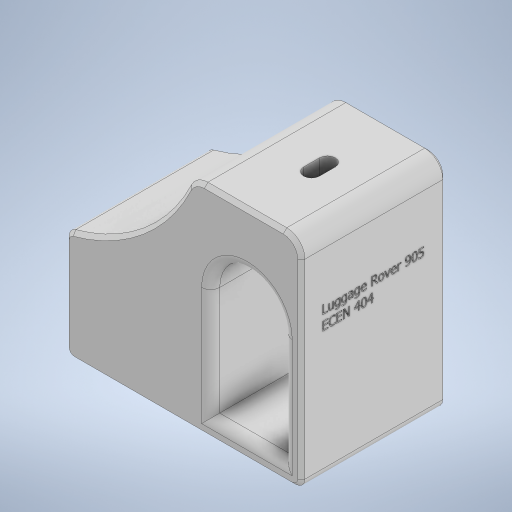
# Autodesk Inventor part: Luggage Mount
Saved by Autodesk Inventor 2023 (Build 270158000, 158)
## iProperties
Created: 2026-02-02
Part Number: Luggage Mount
Material: Generic
Document SubType Name: Modeling
Designer: Matthew
Density: 1 g/cm^3
Appearance: Default
Author: Matthew
Autodesk Inventor part; units mm, degrees
ref_plane "YZ Plane" through (0, 0, 0) normal (1, 0, 0) x (0, 1, 0)
ref_plane "XZ Plane" through (0, 0, 0) normal (0, 1, 0) x (-1, 0, 0)
ref_plane "XY Plane" through (0, 0, 0) normal (0, 0, 1) x (1, 0, 0)
sketch "Sketch1" plane through (0, 0, 0) normal (0, 0, 1) x (1, 0, 0)
  line L0 (0, 3.175) -> (0, 69.85)
  line L1 (-6.35, 76.2) -> (-19.05, 76.2)
  line L2 (-19.05, 76.2) -> (-19.05, 136.2183)
  line L3 (-19.05, 76.2) -> (-33.9583, 76.2)
  arc A0 (-80.2142, 38.6927) -> (-39.6892, 72.585) centre (-96.9975, 99.9346) ccw
  arc A1 (-33.9583, 76.2) -> (-39.6892, 72.585) centre (-33.9583, 69.85) ccw
  arc A2 (0, 69.85) -> (-6.35, 76.2) centre (-6.35, 69.85) ccw
  arc A3 (-3.175, 0) -> (0, 3.175) centre (-3.175, 3.175) ccw
  line L4 (-82.55, 35.6306) -> (-82.55, 3.175)
  line L5 (-3.175, 0) -> (-79.375, 0)
  arc A4 (-82.55, 3.175) -> (-79.375, 0) centre (-79.375, 3.175) ccw
  arc A5 (-80.2142, 38.6927) -> (-82.55, 35.6306) centre (-79.375, 35.6306) ccw
  point P0 (0, 0)
  point P1 (0, 76.2)
  point P2 (-38.1, 76.2)
  point P3 (-82.55, 38.1)
  dimension "d2" = 19.05
  dimension "d3" = 19.05
  dimension "d6" = 6.35
  dimension "d7" = 3.175
  dimension "d44" = 3.175
  constraints: 14 point on circle, 12 end point, 9 tangent, 6 centre point, 5 point on line, 3 perpendicular, 2 equal radius, 1 horizontal
  measures "d2" distance of point (0, 76.2) L1.end
  measures "d3" distance of L1.end point (-38.1, 76.2)
  measures "d6" radius of A1
  measures "d7" radius of A3
  measures "d44" radius of A4
extrude "Extrusion1" add sketch "Sketch1" along normal blind 50.8
sketch "Sketch5" plane through (0, 0, 50.8) normal (0, 0, 1) x (1, 0, 0)
  line L0 (0, 3.175) -> (0, 69.85) projected
  line L1 (0, 31.4722) -> (19.05, 31.4722) construction
  line L2 (-19.05, 0) -> (-12.7, 0) construction
  line L3 (-19.05, 6.35) -> (-6.35, 6.35)
  line L4 (-19.05, 6.35) -> (-23.1501, 6.35)
  line L5 (-19.05, 6.35) -> (-31.75, 6.35)
  line L6 (-6.35, 6.35) -> (-6.35, 44.45)
  arc A0 (-6.35, 44.45) -> (-19.05, 57.15) centre (-19.05, 44.45) ccw
  line L7 (-31.75, 44.45) -> (-31.75, 6.35)
  arc A1 (-19.05, 57.15) -> (-31.75, 44.45) centre (-19.05, 44.45) ccw
  arc A2 (-33.9583, 76.2) -> (-39.6892, 72.585) centre (-33.9583, 69.85) ccw projected
  arc A3 (-80.2142, 38.6927) -> (-39.6892, 72.585) centre (-96.9975, 99.9346) ccw projected
  arc A4 (-3.175, 0) -> (0, 3.175) centre (-3.175, 3.175) ccw projected
  line L8 (0, 3.175) -> (0, 69.85) projected
  arc A5 (0, 69.85) -> (-6.35, 76.2) centre (-6.35, 69.85) ccw projected
  line L9 (-6.35, 76.2) -> (-33.9583, 76.2) projected
  line L10 (-33.9583, 69.85) -> (-6.35, 69.85)
  line L11 (-6.35, 6.35) -> (-116.693, 6.35)
  arc A6 (-81.1052, 31.9165) -> (-116.693, 6.35) centre (-68.1025, -23.7346) ccw
  arc A7 (-80.2142, 38.6927) -> (-82.55, 35.6306) centre (-79.375, 35.6306) ccw projected
  line L12 (-82.55, 35.6306) -> (-82.55, 3.175) projected
  arc A8 (-82.55, 3.175) -> (-79.375, 0) centre (-79.375, 3.175) ccw projected
  line L13 (-79.375, 0) -> (-3.175, 0) projected
  point P0 (0, 0)
  constraints: 18 end point, 6 point on circle, 3 centre point, 3 horizontal, 1 concentric, 1 perpendicular, 1 point on line
extrude "Extrusion2" cut sketch "Sketch5" against normal blind 50.8 contours L4 L5 L7 A1 A0 L6 L3
fillet "Fillet1" radius 3.175 8 edges at (-6.35, 25.4, 50.8) (-31.75, 25.4, 50.8) (-19.05, 57.15, 50.8) (-31.75, 25.4, 0) (-6.35, 25.4, 0) (-19.05, 57.15, 0) (-19.05, 6.35, 50.8) (-19.05, 6.35, 0)
chamfer "Chamfer1" distance 1.27 angle 45 28 edges at (-20.1542, 76.2, 50.8) (-37.3462, 75.2207, 50.8) (-56.2597, 51.2244, 50.8) (-0.9299, 0.9299, 50.8) (0, 36.5125, 50.8) (-1.8599, 74.3401, 50.8) (-81.8994, 37.5563, 50.8) (-82.55, 19.4028, 50.8) (-81.6201, 0.9299, 50.8) (-41.275, 0, 50.8) (-3.175, 23.8125, 50.8) (-19.05, 3.175, 50.8) (-19.05, 60.325, 50.8) (-34.925, 23.8125, 50.8) (-20.1542, 76.2, 0) (-37.3462, 75.2207, 0) (-56.2597, 51.2244, 0) (-3.175, 23.8125, 0) (-19.05, 3.175, 0) (-19.05, 60.325, 0) (-34.925, 23.8125, 0) (-0.9299, 0.9299, 0) (0, 36.5125, 0) (-1.8599, 74.3401, 0) (-81.8994, 37.5563, 0) (-82.55, 19.4028, 0) (-81.6201, 0.9299, 0) (-41.275, 0, 0)
sketch "Sketch8" plane through (-79.375, 0, 1.27) normal (0, -1, 0) x (1, 0, 0)
  line L0 (79.375, 0) -> (79.375, 48.26) projected
  arc A0 (63.1038, 26.9088) -> (57.5462, 26.9088) centre (60.325, 26.9088) ccw
  arc A1 (57.5462, 21.3512) -> (63.1038, 21.3512) centre (60.325, 21.3512) ccw
  line L1 (57.5462, 21.3512) -> (57.5462, 26.9088)
  line L2 (63.1038, 21.3512) -> (63.1038, 26.9088)
  point P0 (79.375, -1.27)
  constraints: 4 end point, 4 point on circle, 4 tangent, 2 centre point
extrude "Extrusion4" cut sketch "Sketch8" against normal blind 25.4
sketch "Sketch9" plane through (0, 3.175, 1.27) normal (1, 0, 0) x (0, 0, -1)
  line L0 (-42.3879, 49.807) -> (-4.4919, 49.807) construction
  line L1 (-4.4919, 49.807) -> (-4.4919, 26.5095) construction
  line L2 (-4.4919, 26.5095) -> (-42.3879, 26.5095) construction
  line L3 (-42.3879, 26.5095) -> (-42.3879, 49.807) construction
  line L4 (-40.3131, 46.6973) -> (-42.0791, 46.6973)
  line L5 (-42.0791, 46.6973) -> (-42.0791, 49.7453)
  line L6 (-42.0791, 49.7453) -> (-41.6741, 49.7453)
  line L7 (-41.6741, 49.7453) -> (-41.6741, 47.0579)
  line L8 (-41.6741, 47.0579) -> (-40.3131, 47.0579)
  line L9 (-40.3131, 47.0579) -> (-40.3131, 46.6973)
  line L10 (-38.2457, 46.6973) -> (-38.631, 46.6973)
  line L11 (-38.631, 46.6973) -> (-38.631, 46.9492)
  spline S0 degree 2 poles (-38.631, 46.9492) (-38.8088, 46.7936) (-39.1275, 46.6331) (-39.3251, 46.6331) knots 0 0 0 1 2 2 2
  spline S1 degree 2 poles (-39.3251, 46.6331) (-39.4733, 46.6331) (-39.7376, 46.7319) (-39.8339, 46.8381) knots 0 0 0 1 2 2 2
  spline S2 degree 2 poles (-39.8339, 46.8381) (-39.9327, 46.9443) (-40.0414, 47.2678) (-40.0414, 47.5) knots 0 0 0 1 2 2 2
  line L12 (-40.0414, 47.5) -> (-40.0414, 48.9845)
  line L13 (-40.0414, 48.9845) -> (-39.6561, 48.9845)
  line L14 (-39.6561, 48.9845) -> (-39.6561, 47.6803)
  spline S3 degree 2 poles (-39.6561, 47.6803) (-39.6561, 47.4976) (-39.6289, 47.258) (-39.582, 47.169) knots 0 0 0 1 2 2 2
  spline S4 degree 2 poles (-39.582, 47.169) (-39.535, 47.0801) (-39.3745, 46.9986) (-39.2238, 46.9986) knots 0 0 0 1 2 2 2
  spline S5 degree 2 poles (-39.2238, 46.9986) (-39.083, 46.9986) (-38.7644, 47.1592) (-38.631, 47.2753) knots 0 0 0 1 2 2 2
  line L15 (-38.631, 47.2753) -> (-38.631, 48.9845)
  line L16 (-38.631, 48.9845) -> (-38.2457, 48.9845)
  line L17 (-38.2457, 48.9845) -> (-38.2457, 46.6973)
  spline S6 degree 2 poles (-37.6059, 46.3317) (-37.5664, 46.3144) (-37.4158, 46.2601) (-37.3194, 46.2379) knots 0 0 0 1 2 2 2
  spline S7 degree 2 poles (-37.3194, 46.2379) (-37.2132, 46.2107) (-37.0329, 46.1786) (-36.9267, 46.1786) knots 0 0 0 1 2 2 2
  spline S8 degree 2 poles (-36.9267, 46.1786) (-36.7489, 46.1786) (-36.5018, 46.2724) (-36.4327, 46.3564) knots 0 0 0 1 2 2 2
  spline S9 degree 2 poles (-36.4327, 46.3564) (-36.366, 46.4404) (-36.3141, 46.6602) (-36.3141, 46.801) knots 0 0 0 1 2 2 2
  line L18 (-36.3141, 46.801) -> (-36.3141, 47.0011)
  spline S10 degree 2 poles (-36.3141, 47.0011) (-36.4697, 46.8652) (-36.7686, 46.7368) (-36.9934, 46.7368) knots 0 0 0 1 2 2 2
  spline S11 degree 2 poles (-36.9934, 46.7368) (-37.3836, 46.7368) (-37.8455, 47.3173) (-37.8455, 47.8631) knots 0 0 0 1 2 2 2
  spline S12 degree 2 poles (-37.8455, 47.8631) (-37.8455, 48.1472) (-37.685, 48.5868) (-37.5516, 48.7424) knots 0 0 0 1 2 2 2
  spline S13 degree 2 poles (-37.5516, 48.7424) (-37.4232, 48.8882) (-37.07, 49.0487) (-36.8822, 49.0487) knots 0 0 0 1 2 2 2
  spline S14 degree 2 poles (-36.8822, 49.0487) (-36.7044, 49.0487) (-36.445, 48.9648) (-36.3141, 48.8882) knots 0 0 0 1 2 2 2
  line L19 (-36.3141, 48.8882) -> (-36.2919, 48.9845)
  line L20 (-36.2919, 48.9845) -> (-35.9288, 48.9845)
  line L21 (-35.9288, 48.9845) -> (-35.9288, 46.9591)
  spline S15 degree 2 poles (-35.9288, 46.9591) (-35.9288, 46.3762) (-36.4352, 45.8328) (-36.9563, 45.8328) knots 0 0 0 1 2 2 2
  spline S16 degree 2 poles (-36.9563, 45.8328) (-37.1243, 45.8328) (-37.475, 45.8871) (-37.6257, 45.9316) knots 0 0 0 1 2 2 2
  line L22 (-37.6257, 45.9316) -> (-37.6257, 46.3317)
  line L23 (-37.6257, 46.3317) -> (-37.6059, 46.3317)
  line L24 (-36.3141, 47.3173) -> (-36.3141, 48.5745)
  spline S17 degree 2 poles (-36.3141, 48.5745) (-36.4574, 48.6436) (-36.6995, 48.7029) (-36.8205, 48.7029) knots 0 0 0 1 2 2 2
  spline S18 degree 2 poles (-36.8205, 48.7029) (-37.1119, 48.7029) (-37.4479, 48.2731) (-37.4479, 47.8705) knots 0 0 0 1 2 2 2
  spline S19 degree 2 poles (-37.4479, 47.8705) (-37.4479, 47.4902) (-37.1935, 47.0925) (-36.9069, 47.0925) knots 0 0 0 1 2 2 2
  spline S20 degree 2 poles (-36.9069, 47.0925) (-36.7563, 47.0925) (-36.4401, 47.211) (-36.3141, 47.3173) knots 0 0 0 1 2 2 2
  spline S21 degree 2 poles (-35.2891, 46.3317) (-35.2496, 46.3144) (-35.0989, 46.2601) (-35.0025, 46.2379) knots 0 0 0 1 2 2 2
  spline S22 degree 2 poles (-35.0025, 46.2379) (-34.8963, 46.2107) (-34.716, 46.1786) (-34.6098, 46.1786) knots 0 0 0 1 2 2 2
  spline S23 degree 2 poles (-34.6098, 46.1786) (-34.432, 46.1786) (-34.185, 46.2724) (-34.1158, 46.3564) knots 0 0 0 1 2 2 2
  spline S24 degree 2 poles (-34.1158, 46.3564) (-34.0491, 46.4404) (-33.9973, 46.6602) (-33.9973, 46.801) knots 0 0 0 1 2 2 2
  line L25 (-33.9973, 46.801) -> (-33.9973, 47.0011)
  spline S25 degree 2 poles (-33.9973, 47.0011) (-34.1529, 46.8652) (-34.4517, 46.7368) (-34.6765, 46.7368) knots 0 0 0 1 2 2 2
  spline S26 degree 2 poles (-34.6765, 46.7368) (-35.0668, 46.7368) (-35.5287, 47.3173) (-35.5287, 47.8631) knots 0 0 0 1 2 2 2
  spline S27 degree 2 poles (-35.5287, 47.8631) (-35.5287, 48.1472) (-35.3681, 48.5868) (-35.2347, 48.7424) knots 0 0 0 1 2 2 2
  spline S28 degree 2 poles (-35.2347, 48.7424) (-35.1063, 48.8882) (-34.7531, 49.0487) (-34.5654, 49.0487) knots 0 0 0 1 2 2 2
  spline S29 degree 2 poles (-34.5654, 49.0487) (-34.3875, 49.0487) (-34.1282, 48.9648) (-33.9973, 48.8882) knots 0 0 0 1 2 2 2
  line L26 (-33.9973, 48.8882) -> (-33.975, 48.9845)
  line L27 (-33.975, 48.9845) -> (-33.6119, 48.9845)
  line L28 (-33.6119, 48.9845) -> (-33.6119, 46.9591)
  spline S30 degree 2 poles (-33.6119, 46.9591) (-33.6119, 46.3762) (-34.1183, 45.8328) (-34.6395, 45.8328) knots 0 0 0 1 2 2 2
  spline S31 degree 2 poles (-34.6395, 45.8328) (-34.8074, 45.8328) (-35.1582, 45.8871) (-35.3088, 45.9316) knots 0 0 0 1 2 2 2
  line L29 (-35.3088, 45.9316) -> (-35.3088, 46.3317)
  line L30 (-35.3088, 46.3317) -> (-35.2891, 46.3317)
  line L31 (-33.9973, 47.3173) -> (-33.9973, 48.5745)
  spline S32 degree 2 poles (-33.9973, 48.5745) (-34.1405, 48.6436) (-34.3826, 48.7029) (-34.5036, 48.7029) knots 0 0 0 1 2 2 2
  spline S33 degree 2 poles (-34.5036, 48.7029) (-34.7951, 48.7029) (-35.131, 48.2731) (-35.131, 47.8705) knots 0 0 0 1 2 2 2
  spline S34 degree 2 poles (-35.131, 47.8705) (-35.131, 47.4902) (-34.8766, 47.0925) (-34.5901, 47.0925) knots 0 0 0 1 2 2 2
  spline S35 degree 2 poles (-34.5901, 47.0925) (-34.4394, 47.0925) (-34.1232, 47.211) (-33.9973, 47.3173) knots 0 0 0 1 2 2 2
  spline S36 degree 2 poles (-31.7792, 46.9393) (-31.8261, 46.9048) (-31.9842, 46.7813) (-32.0583, 46.7442) knots 0 0 0 1 2 2 2
  spline S37 degree 2 poles (-32.0583, 46.7442) (-32.1596, 46.6899) (-32.3498, 46.6331) (-32.5227, 46.6331) knots 0 0 0 1 2 2 2
  spline S38 degree 2 poles (-32.5227, 46.6331) (-32.6634, 46.6331) (-32.9179, 46.7393) (-33.0142, 46.8356) knots 0 0 0 1 2 2 2
  spline S39 degree 2 poles (-33.0142, 46.8356) (-33.1056, 46.9295) (-33.2167, 47.2061) (-33.2167, 47.3592) knots 0 0 0 1 2 2 2
  spline S40 degree 2 poles (-33.2167, 47.3592) (-33.2167, 47.5964) (-33.0167, 47.9323) (-32.7993, 48.0286) knots 0 0 0 1 2 2 2
  spline S41 degree 2 poles (-32.7993, 48.0286) (-32.6066, 48.1175) (-32.083, 48.1842) (-31.7792, 48.2015) knots 0 0 0 1 2 2 2
  line L32 (-31.7792, 48.2015) -> (-31.7792, 48.2756)
  spline S42 degree 2 poles (-31.7792, 48.2756) (-31.7792, 48.409) (-31.8607, 48.5745) (-31.9348, 48.6214) knots 0 0 0 1 2 2 2
  spline S43 degree 2 poles (-31.9348, 48.6214) (-32.0089, 48.6683) (-32.2213, 48.698) (-32.3349, 48.698) knots 0 0 0 1 2 2 2
  spline S44 degree 2 poles (-32.3349, 48.698) (-32.4683, 48.698) (-32.8289, 48.6189) (-33.0092, 48.5424) knots 0 0 0 1 2 2 2
  line L33 (-33.0092, 48.5424) -> (-33.0315, 48.5424)
  line L34 (-33.0315, 48.5424) -> (-33.0315, 48.9351)
  spline S45 degree 2 poles (-33.0315, 48.9351) (-32.9253, 48.9648) (-32.5276, 49.0389) (-32.3325, 49.0389) knots 0 0 0 1 2 2 2
  spline S46 degree 2 poles (-32.3325, 49.0389) (-32.0953, 49.0389) (-31.7718, 48.9648) (-31.6433, 48.8684) knots 0 0 0 1 2 2 2
  spline S47 degree 2 poles (-31.6433, 48.8684) (-31.5174, 48.7746) (-31.3939, 48.4757) (-31.3939, 48.2608) knots 0 0 0 1 2 2 2
  line L35 (-31.3939, 48.2608) -> (-31.3939, 46.6973)
  line L36 (-31.3939, 46.6973) -> (-31.7792, 46.6973)
  line L37 (-31.7792, 46.6973) -> (-31.7792, 46.9393)
  line L38 (-31.7792, 47.2604) -> (-31.7792, 47.8952)
  spline S48 degree 2 poles (-31.7792, 47.8952) (-31.9175, 47.8829) (-32.3349, 47.8409) (-32.4658, 47.8014) knots 0 0 0 1 2 2 2
  spline S49 degree 2 poles (-32.4658, 47.8014) (-32.619, 47.7544) (-32.8191, 47.5593) (-32.8191, 47.3864) knots 0 0 0 1 2 2 2
  spline S50 degree 2 poles (-32.8191, 47.3864) (-32.8191, 47.1888) (-32.5968, 46.9887) (-32.3843, 46.9887) knots 0 0 0 1 2 2 2
  spline S51 degree 2 poles (-32.3843, 46.9887) (-32.204, 46.9887) (-31.9076, 47.1443) (-31.7792, 47.2604) knots 0 0 0 1 2 2 2
  spline S52 degree 2 poles (-30.7714, 46.3317) (-30.7319, 46.3144) (-30.5812, 46.2601) (-30.4849, 46.2379) knots 0 0 0 1 2 2 2
  spline S53 degree 2 poles (-30.4849, 46.2379) (-30.3787, 46.2107) (-30.1984, 46.1786) (-30.0922, 46.1786) knots 0 0 0 1 2 2 2
  spline S54 degree 2 poles (-30.0922, 46.1786) (-29.9143, 46.1786) (-29.6673, 46.2724) (-29.5982, 46.3564) knots 0 0 0 1 2 2 2
  spline S55 degree 2 poles (-29.5982, 46.3564) (-29.5315, 46.4404) (-29.4796, 46.6602) (-29.4796, 46.801) knots 0 0 0 1 2 2 2
  line L39 (-29.4796, 46.801) -> (-29.4796, 47.0011)
  spline S56 degree 2 poles (-29.4796, 47.0011) (-29.6352, 46.8652) (-29.9341, 46.7368) (-30.1588, 46.7368) knots 0 0 0 1 2 2 2
  spline S57 degree 2 poles (-30.1588, 46.7368) (-30.5491, 46.7368) (-31.011, 47.3173) (-31.011, 47.8631) knots 0 0 0 1 2 2 2
  spline S58 degree 2 poles (-31.011, 47.8631) (-31.011, 48.1472) (-30.8505, 48.5868) (-30.7171, 48.7424) knots 0 0 0 1 2 2 2
  spline S59 degree 2 poles (-30.7171, 48.7424) (-30.5886, 48.8882) (-30.2354, 49.0487) (-30.0477, 49.0487) knots 0 0 0 1 2 2 2
  spline S60 degree 2 poles (-30.0477, 49.0487) (-29.8699, 49.0487) (-29.6105, 48.9648) (-29.4796, 48.8882) knots 0 0 0 1 2 2 2
  line L40 (-29.4796, 48.8882) -> (-29.4574, 48.9845)
  line L41 (-29.4574, 48.9845) -> (-29.0943, 48.9845)
  line L42 (-29.0943, 48.9845) -> (-29.0943, 46.9591)
  spline S61 degree 2 poles (-29.0943, 46.9591) (-29.0943, 46.3762) (-29.6006, 45.8328) (-30.1218, 45.8328) knots 0 0 0 1 2 2 2
  spline S62 degree 2 poles (-30.1218, 45.8328) (-30.2898, 45.8328) (-30.6405, 45.8871) (-30.7912, 45.9316) knots 0 0 0 1 2 2 2
  line L43 (-30.7912, 45.9316) -> (-30.7912, 46.3317)
  line L44 (-30.7912, 46.3317) -> (-30.7714, 46.3317)
  line L45 (-29.4796, 47.3173) -> (-29.4796, 48.5745)
  spline S63 degree 2 poles (-29.4796, 48.5745) (-29.6229, 48.6436) (-29.8649, 48.7029) (-29.9859, 48.7029) knots 0 0 0 1 2 2 2
  spline S64 degree 2 poles (-29.9859, 48.7029) (-30.2774, 48.7029) (-30.6133, 48.2731) (-30.6133, 47.8705) knots 0 0 0 1 2 2 2
  spline S65 degree 2 poles (-30.6133, 47.8705) (-30.6133, 47.4902) (-30.3589, 47.0925) (-30.0724, 47.0925) knots 0 0 0 1 2 2 2
  spline S66 degree 2 poles (-30.0724, 47.0925) (-29.9217, 47.0925) (-29.6056, 47.211) (-29.4796, 47.3173) knots 0 0 0 1 2 2 2
  spline S67 degree 2 poles (-27.5431, 46.6454) (-28.0914, 46.6454) (-28.6941, 47.2604) (-28.6941, 47.8285) knots 0 0 0 1 2 2 2
  spline S68 degree 2 poles (-28.6941, 47.8285) (-28.6941, 48.3868) (-28.1087, 49.0487) (-27.637, 49.0487) knots 0 0 0 1 2 2 2
  spline S69 degree 2 poles (-27.637, 49.0487) (-27.4245, 49.0487) (-27.096, 48.9252) (-26.975, 48.7943) knots 0 0 0 1 2 2 2
  spline S70 degree 2 poles (-26.975, 48.7943) (-26.8515, 48.6634) (-26.7206, 48.2855) (-26.7206, 48.0113) knots 0 0 0 1 2 2 2
  line L46 (-26.7206, 48.0113) -> (-26.7206, 47.8014)
  line L47 (-26.7206, 47.8014) -> (-28.3039, 47.8014)
  spline S71 degree 2 poles (-28.3039, 47.8014) (-28.3039, 47.4037) (-27.9037, 46.9813) (-27.548, 46.9813) knots 0 0 0 1 2 2 2
  spline S72 degree 2 poles (-27.548, 46.9813) (-27.4221, 46.9813) (-27.1775, 47.0381) (-27.0787, 47.0826) knots 0 0 0 1 2 2 2
  spline S73 degree 2 poles (-27.0787, 47.0826) (-26.975, 47.132) (-26.8317, 47.2184) (-26.7848, 47.258) knots 0 0 0 1 2 2 2
  line L48 (-26.7848, 47.258) -> (-26.7626, 47.258)
  line L49 (-26.7626, 47.258) -> (-26.7626, 46.8381)
  spline S74 degree 2 poles (-26.7626, 46.8381) (-26.8293, 46.8109) (-27.0318, 46.7319) (-27.1108, 46.7096) knots 0 0 0 1 2 2 2
  spline S75 degree 2 poles (-27.1108, 46.7096) (-27.222, 46.6775) (-27.4048, 46.6454) (-27.5431, 46.6454) knots 0 0 0 1 2 2 2
  spline S76 degree 2 poles (-27.096, 48.0953) (-27.101, 48.2509) (-27.1652, 48.4782) (-27.2269, 48.5547) knots 0 0 0 1 2 2 2
  spline S77 degree 2 poles (-27.2269, 48.5547) (-27.2936, 48.6412) (-27.5036, 48.7326) (-27.6592, 48.7326) knots 0 0 0 1 2 2 2
  spline S78 degree 2 poles (-27.6592, 48.7326) (-27.8123, 48.7326) (-28.0272, 48.6412) (-28.1161, 48.5523) knots 0 0 0 1 2 2 2
  spline S79 degree 2 poles (-28.1161, 48.5523) (-28.2026, 48.4609) (-28.2915, 48.241) (-28.3039, 48.0953) knots 0 0 0 1 2 2 2
  line L50 (-28.3039, 48.0953) -> (-27.096, 48.0953)
  line L51 (-22.6327, 46.6973) -> (-23.1588, 46.6973)
  line L52 (-23.1588, 46.6973) -> (-24.1221, 47.9101)
  line L53 (-24.1221, 47.9101) -> (-24.5865, 47.9101)
  line L54 (-24.5865, 47.9101) -> (-24.5865, 46.6973)
  line L55 (-24.5865, 46.6973) -> (-24.9916, 46.6973)
  line L56 (-24.9916, 46.6973) -> (-24.9916, 49.7453)
  line L57 (-24.9916, 49.7453) -> (-24.2061, 49.7453)
  spline S80 degree 2 poles (-24.2061, 49.7453) (-23.9443, 49.7453) (-23.5911, 49.6885) (-23.4305, 49.5847) knots 0 0 0 1 2 2 2
  spline S81 degree 2 poles (-23.4305, 49.5847) (-23.27, 49.481) (-23.0847, 49.1574) (-23.0847, 48.9178) knots 0 0 0 1 2 2 2
  spline S82 degree 2 poles (-23.0847, 48.9178) (-23.0847, 48.5844) (-23.4256, 48.1324) (-23.717, 48.0237) knots 0 0 0 1 2 2 2
  line L58 (-23.717, 48.0237) -> (-22.6327, 46.6973)
  spline S83 degree 2 poles (-23.5071, 48.8857) (-23.5071, 49.0191) (-23.601, 49.2241) (-23.6998, 49.2908) knots 0 0 0 1 2 2 2
  spline S84 degree 2 poles (-23.6998, 49.2908) (-23.7862, 49.3476) (-24.0159, 49.3945) (-24.1839, 49.3945) knots 0 0 0 1 2 2 2
  line L59 (-24.1839, 49.3945) -> (-24.5865, 49.3945)
  line L60 (-24.5865, 49.3945) -> (-24.5865, 48.2484)
  line L61 (-24.5865, 48.2484) -> (-24.2308, 48.2484)
  spline S85 degree 2 poles (-24.2308, 48.2484) (-24.0554, 48.2484) (-23.7763, 48.3102) (-23.68, 48.4065) knots 0 0 0 1 2 2 2
  spline S86 degree 2 poles (-23.68, 48.4065) (-23.5911, 48.4905) (-23.5071, 48.7276) (-23.5071, 48.8857) knots 0 0 0 1 2 2 2
  spline S87 degree 2 poles (-20.5406, 47.8409) (-20.5406, 47.2629) (-21.0964, 46.6331) (-21.5607, 46.6331) knots 0 0 0 1 2 2 2
  spline S88 degree 2 poles (-21.5607, 46.6331) (-22.0374, 46.6331) (-22.5833, 47.2827) (-22.5833, 47.8409) knots 0 0 0 1 2 2 2
  spline S89 degree 2 poles (-22.5833, 47.8409) (-22.5833, 48.4139) (-22.0201, 49.0487) (-21.5607, 49.0487) knots 0 0 0 1 2 2 2
  spline S90 degree 2 poles (-21.5607, 49.0487) (-21.0964, 49.0487) (-20.5406, 48.4164) (-20.5406, 47.8409) knots 0 0 0 1 2 2 2
  spline S91 degree 2 poles (-20.9383, 47.8409) (-20.9383, 48.2855) (-21.2618, 48.7177) (-21.5607, 48.7177) knots 0 0 0 1 2 2 2
  spline S92 degree 2 poles (-21.5607, 48.7177) (-21.8596, 48.7177) (-22.1856, 48.2855) (-22.1856, 47.8409) knots 0 0 0 1 2 2 2
  spline S93 degree 2 poles (-22.1856, 47.8409) (-22.1856, 47.4086) (-21.8596, 46.964) (-21.5607, 46.964) knots 0 0 0 1 2 2 2
  spline S94 degree 2 poles (-21.5607, 46.964) (-21.2643, 46.964) (-20.9383, 47.4012) (-20.9383, 47.8409) knots 0 0 0 1 2 2 2
  line L62 (-18.3497, 48.9845) -> (-19.2117, 46.6973)
  line L63 (-19.2117, 46.6973) -> (-19.5575, 46.6973)
  line L64 (-19.5575, 46.6973) -> (-20.4122, 48.9845)
  line L65 (-20.4122, 48.9845) -> (-19.9947, 48.9845)
  line L66 (-19.9947, 48.9845) -> (-19.3698, 47.2234)
  line L67 (-19.3698, 47.2234) -> (-18.7498, 48.9845)
  line L68 (-18.7498, 48.9845) -> (-18.3497, 48.9845)
  spline S95 degree 2 poles (-17.0653, 46.6454) (-17.6136, 46.6454) (-18.2163, 47.2604) (-18.2163, 47.8285) knots 0 0 0 1 2 2 2
  spline S96 degree 2 poles (-18.2163, 47.8285) (-18.2163, 48.3868) (-17.6309, 49.0487) (-17.1592, 49.0487) knots 0 0 0 1 2 2 2
  spline S97 degree 2 poles (-17.1592, 49.0487) (-16.9467, 49.0487) (-16.6182, 48.9252) (-16.4972, 48.7943) knots 0 0 0 1 2 2 2
  spline S98 degree 2 poles (-16.4972, 48.7943) (-16.3737, 48.6634) (-16.2428, 48.2855) (-16.2428, 48.0113) knots 0 0 0 1 2 2 2
  line L69 (-16.2428, 48.0113) -> (-16.2428, 47.8014)
  line L70 (-16.2428, 47.8014) -> (-17.8261, 47.8014)
  spline S99 degree 2 poles (-17.8261, 47.8014) (-17.8261, 47.4037) (-17.4259, 46.9813) (-17.0702, 46.9813) knots 0 0 0 1 2 2 2
  spline S100 degree 2 poles (-17.0702, 46.9813) (-16.9443, 46.9813) (-16.6997, 47.0381) (-16.6009, 47.0826) knots 0 0 0 1 2 2 2
  spline S101 degree 2 poles (-16.6009, 47.0826) (-16.4972, 47.132) (-16.3539, 47.2184) (-16.307, 47.258) knots 0 0 0 1 2 2 2
  line L71 (-16.307, 47.258) -> (-16.2848, 47.258)
  line L72 (-16.2848, 47.258) -> (-16.2848, 46.8381)
  spline S102 degree 2 poles (-16.2848, 46.8381) (-16.3515, 46.8109) (-16.554, 46.7319) (-16.633, 46.7096) knots 0 0 0 1 2 2 2
  spline S103 degree 2 poles (-16.633, 46.7096) (-16.7442, 46.6775) (-16.927, 46.6454) (-17.0653, 46.6454) knots 0 0 0 1 2 2 2
  spline S104 degree 2 poles (-16.6182, 48.0953) (-16.6232, 48.2509) (-16.6874, 48.4782) (-16.7491, 48.5547) knots 0 0 0 1 2 2 2
  spline S105 degree 2 poles (-16.7491, 48.5547) (-16.8158, 48.6412) (-17.0258, 48.7326) (-17.1814, 48.7326) knots 0 0 0 1 2 2 2
  spline S106 degree 2 poles (-17.1814, 48.7326) (-17.3345, 48.7326) (-17.5494, 48.6412) (-17.6383, 48.5523) knots 0 0 0 1 2 2 2
  spline S107 degree 2 poles (-17.6383, 48.5523) (-17.7248, 48.4609) (-17.8137, 48.241) (-17.8261, 48.0953) knots 0 0 0 1 2 2 2
  line L73 (-17.8261, 48.0953) -> (-16.6182, 48.0953)
  line L74 (-14.6397, 48.572) -> (-14.6595, 48.572)
  spline S108 degree 2 poles (-14.6595, 48.572) (-14.704, 48.5844) (-14.8003, 48.5893) (-14.867, 48.5893) knots 0 0 0 1 2 2 2
  spline S109 degree 2 poles (-14.867, 48.5893) (-15.0226, 48.5893) (-15.3289, 48.4535) (-15.4672, 48.3201) knots 0 0 0 1 2 2 2
  line L75 (-15.4672, 48.3201) -> (-15.4672, 46.6973)
  line L76 (-15.4672, 46.6973) -> (-15.8525, 46.6973)
  line L77 (-15.8525, 46.6973) -> (-15.8525, 48.9845)
  line L78 (-15.8525, 48.9845) -> (-15.4672, 48.9845)
  line L79 (-15.4672, 48.9845) -> (-15.4672, 48.6436)
  spline S110 degree 2 poles (-15.4672, 48.6436) (-15.2572, 48.8314) (-14.9435, 48.9845) (-14.7953, 48.9845) knots 0 0 0 1 2 2 2
  spline S111 degree 2 poles (-14.7953, 48.9845) (-14.7361, 48.9845) (-14.6768, 48.9796) (-14.6397, 48.9722) knots 0 0 0 1 2 2 2
  line L80 (-14.6397, 48.9722) -> (-14.6397, 48.572)
  spline S112 degree 2 poles (-13.1725, 48.7548) (-13.1725, 48.9895) (-13.0194, 49.3797) (-12.886, 49.5205) knots 0 0 0 1 2 2 2
  spline S113 degree 2 poles (-12.886, 49.5205) (-12.7601, 49.6564) (-12.392, 49.807) (-12.2043, 49.807) knots 0 0 0 1 2 2 2
  spline S114 degree 2 poles (-12.2043, 49.807) (-11.9943, 49.807) (-11.6535, 49.6662) (-11.5275, 49.5329) knots 0 0 0 1 2 2 2
  spline S115 degree 2 poles (-11.5275, 49.5329) (-11.3694, 49.3649) (-11.1965, 48.8215) (-11.1965, 48.4041) knots 0 0 0 1 2 2 2
  spline S116 degree 2 poles (-11.1965, 48.4041) (-11.1965, 48.0261) (-11.367, 47.3494) (-11.5325, 47.1246) knots 0 0 0 1 2 2 2
  spline S117 degree 2 poles (-11.5325, 47.1246) (-11.7078, 46.8875) (-12.2018, 46.638) (-12.5625, 46.638) knots 0 0 0 1 2 2 2
  spline S118 degree 2 poles (-12.5625, 46.638) (-12.644, 46.638) (-12.8292, 46.6553) (-12.9083, 46.68) knots 0 0 0 1 2 2 2
  line L81 (-12.9083, 46.68) -> (-12.9083, 47.0727)
  line L82 (-12.9083, 47.0727) -> (-12.8885, 47.0727)
  spline S119 degree 2 poles (-12.8885, 47.0727) (-12.8366, 47.0431) (-12.6193, 46.9912) (-12.5081, 46.9912) knots 0 0 0 1 2 2 2
  spline S120 degree 2 poles (-12.5081, 46.9912) (-12.108, 46.9912) (-11.651, 47.5198) (-11.6189, 48.0089) knots 0 0 0 1 2 2 2
  spline S121 degree 2 poles (-11.6189, 48.0089) (-11.7819, 47.8977) (-12.0783, 47.7964) (-12.2537, 47.7964) knots 0 0 0 1 2 2 2
  spline S122 degree 2 poles (-12.2537, 47.7964) (-12.4217, 47.7964) (-12.7008, 47.8705) (-12.8416, 47.9767) knots 0 0 0 1 2 2 2
  spline S123 degree 2 poles (-12.8416, 47.9767) (-13.0046, 48.1027) (-13.1725, 48.4856) (-13.1725, 48.7548) knots 0 0 0 1 2 2 2
  spline S124 degree 2 poles (-11.609, 48.4954) (-11.609, 48.8042) (-11.7226, 49.1945) (-11.8239, 49.3007) knots 0 0 0 1 2 2 2
  spline S125 degree 2 poles (-11.8239, 49.3007) (-11.9128, 49.3995) (-12.0981, 49.4736) (-12.2068, 49.4736) knots 0 0 0 1 2 2 2
  spline S126 degree 2 poles (-12.2068, 49.4736) (-12.4587, 49.4736) (-12.7576, 49.113) (-12.7576, 48.7721) knots 0 0 0 1 2 2 2
  spline S127 degree 2 poles (-12.7576, 48.7721) (-12.7576, 48.5794) (-12.6588, 48.33) (-12.5501, 48.241) knots 0 0 0 1 2 2 2
  spline S128 degree 2 poles (-12.5501, 48.241) (-12.4711, 48.1768) (-12.2759, 48.1348) (-12.1623, 48.1348) knots 0 0 0 1 2 2 2
  spline S129 degree 2 poles (-12.1623, 48.1348) (-12.0314, 48.1348) (-11.7301, 48.2262) (-11.6164, 48.3028) knots 0 0 0 1 2 2 2
  spline S130 degree 2 poles (-11.6164, 48.3028) (-11.614, 48.3324) (-11.609, 48.4337) (-11.609, 48.4954) knots 0 0 0 1 2 2 2
  spline S131 degree 2 poles (-8.9044, 48.2213) (-8.9044, 47.4012) (-9.3811, 46.6331) (-9.8775, 46.6331) knots 0 0 0 1 2 2 2
  spline S132 degree 2 poles (-9.8775, 46.6331) (-10.3814, 46.6331) (-10.8532, 47.4161) (-10.8532, 48.2188) knots 0 0 0 1 2 2 2
  spline S133 degree 2 poles (-10.8532, 48.2188) (-10.8532, 49.0438) (-10.3765, 49.807) (-9.8775, 49.807) knots 0 0 0 1 2 2 2
  spline S134 degree 2 poles (-9.8775, 49.807) (-9.3761, 49.807) (-8.9044, 49.0166) (-8.9044, 48.2213) knots 0 0 0 1 2 2 2
  spline S135 degree 2 poles (-9.428, 47.2925) (-9.3687, 47.4432) (-9.3193, 47.9076) (-9.3193, 48.2213) knots 0 0 0 1 2 2 2
  spline S136 degree 2 poles (-9.3193, 48.2213) (-9.3193, 48.535) (-9.3687, 48.9969) (-9.4305, 49.1525) knots 0 0 0 1 2 2 2
  spline S137 degree 2 poles (-9.4305, 49.1525) (-9.4922, 49.3081) (-9.7071, 49.4686) (-9.8775, 49.4686) knots 0 0 0 1 2 2 2
  spline S138 degree 2 poles (-9.8775, 49.4686) (-10.048, 49.4686) (-10.2678, 49.3081) (-10.332, 49.1475) knots 0 0 0 1 2 2 2
  spline S139 degree 2 poles (-10.332, 49.1475) (-10.3938, 48.9919) (-10.4382, 48.5177) (-10.4382, 48.2188) knots 0 0 0 1 2 2 2
  spline S140 degree 2 poles (-10.4382, 48.2188) (-10.4382, 47.8977) (-10.3987, 47.4679) (-10.3345, 47.3) knots 0 0 0 1 2 2 2
  spline S141 degree 2 poles (-10.3345, 47.3) (-10.2752, 47.1419) (-10.0554, 46.9714) (-9.8775, 46.9714) knots 0 0 0 1 2 2 2
  spline S142 degree 2 poles (-9.8775, 46.9714) (-9.7096, 46.9714) (-9.4898, 47.132) (-9.428, 47.2925) knots 0 0 0 1 2 2 2
  spline S143 degree 2 poles (-6.6665, 47.6655) (-6.6665, 47.4457) (-6.8073, 47.0702) (-6.9358, 46.9319) knots 0 0 0 1 2 2 2
  spline S144 degree 2 poles (-6.9358, 46.9319) (-7.0642, 46.7936) (-7.447, 46.6331) (-7.6842, 46.6331) knots 0 0 0 1 2 2 2
  spline S145 degree 2 poles (-7.6842, 46.6331) (-7.9015, 46.6331) (-8.3264, 46.7294) (-8.482, 46.806) knots 0 0 0 1 2 2 2
  line L83 (-8.482, 46.806) -> (-8.482, 47.2382)
  line L84 (-8.482, 47.2382) -> (-8.4523, 47.2382)
  spline S146 degree 2 poles (-8.4523, 47.2382) (-8.4054, 47.2036) (-8.23, 47.1147) (-8.1238, 47.0752) knots 0 0 0 1 2 2 2
  spline S147 degree 2 poles (-8.1238, 47.0752) (-8.0028, 47.0332) (-7.8027, 46.9863) (-7.6768, 46.9863) knots 0 0 0 1 2 2 2
  spline S148 degree 2 poles (-7.6768, 46.9863) (-7.5533, 46.9863) (-7.3211, 47.0752) (-7.2371, 47.1715) knots 0 0 0 1 2 2 2
  spline S149 degree 2 poles (-7.2371, 47.1715) (-7.1605, 47.2629) (-7.0815, 47.505) (-7.0815, 47.668) knots 0 0 0 1 2 2 2
  spline S150 degree 2 poles (-7.0815, 47.668) (-7.0815, 47.831) (-7.1704, 48.0385) (-7.2544, 48.1077) knots 0 0 0 1 2 2 2
  spline S151 degree 2 poles (-7.2544, 48.1077) (-7.3408, 48.1842) (-7.5977, 48.2484) (-7.7533, 48.2484) knots 0 0 0 1 2 2 2
  spline S152 degree 2 poles (-7.7533, 48.2484) (-7.9213, 48.2484) (-8.2547, 48.1966) (-8.356, 48.1743) knots 0 0 0 1 2 2 2
  line L85 (-8.356, 48.1743) -> (-8.356, 49.7453)
  line L86 (-8.356, 49.7453) -> (-6.6838, 49.7453)
  line L87 (-6.6838, 49.7453) -> (-6.6838, 49.3871)
  line L88 (-6.6838, 49.3871) -> (-7.9633, 49.3871)
  line L89 (-7.9633, 49.3871) -> (-7.9633, 48.5745)
  spline S153 degree 2 poles (-7.9633, 48.5745) (-7.8892, 48.5844) (-7.7459, 48.5918) (-7.6866, 48.5918) knots 0 0 0 1 2 2 2
  spline S154 degree 2 poles (-7.6866, 48.5918) (-7.452, 48.5918) (-7.1284, 48.5152) (-6.9802, 48.4016) knots 0 0 0 1 2 2 2
  spline S155 degree 2 poles (-6.9802, 48.4016) (-6.8295, 48.288) (-6.6665, 47.9422) (-6.6665, 47.6655) knots 0 0 0 1 2 2 2
  line L90 (-42.0791, 41.6788) -> (-42.0791, 44.7268)
  line L91 (-42.0791, 44.7268) -> (-40.1723, 44.7268)
  line L92 (-40.1723, 44.7268) -> (-40.1723, 44.3662)
  line L93 (-40.1723, 44.3662) -> (-41.6741, 44.3662)
  line L94 (-41.6741, 44.3662) -> (-41.6741, 43.5313)
  line L95 (-41.6741, 43.5313) -> (-40.2736, 43.5313)
  line L96 (-40.2736, 43.5313) -> (-40.2736, 43.1707)
  line L97 (-40.2736, 43.1707) -> (-41.6741, 43.1707)
  line L98 (-41.6741, 43.1707) -> (-41.6741, 42.0394)
  line L99 (-41.6741, 42.0394) -> (-40.1723, 42.0394)
  line L100 (-40.1723, 42.0394) -> (-40.1723, 41.6788)
  line L101 (-40.1723, 41.6788) -> (-42.0791, 41.6788)
  spline S156 degree 2 poles (-38.5371, 41.6245) (-38.8335, 41.6245) (-39.335, 41.8246) (-39.5177, 42.0246) knots 0 0 0 1 2 2 2
  spline S157 degree 2 poles (-39.5177, 42.0246) (-39.7005, 42.2222) (-39.9006, 42.815) (-39.9006, 43.2004) knots 0 0 0 1 2 2 2
  spline S158 degree 2 poles (-39.9006, 43.2004) (-39.9006, 43.5832) (-39.7055, 44.1513) (-39.5202, 44.3613) knots 0 0 0 1 2 2 2
  spline S159 degree 2 poles (-39.5202, 44.3613) (-39.3374, 44.5663) (-38.8385, 44.7812) (-38.5297, 44.7812) knots 0 0 0 1 2 2 2
  spline S160 degree 2 poles (-38.5297, 44.7812) (-38.3766, 44.7812) (-38.1074, 44.7367) (-37.9937, 44.7021) knots 0 0 0 1 2 2 2
  spline S161 degree 2 poles (-37.9937, 44.7021) (-37.8949, 44.67) (-37.6899, 44.5786) (-37.5887, 44.5243) knots 0 0 0 1 2 2 2
  line L102 (-37.5887, 44.5243) -> (-37.5887, 44.0352)
  line L103 (-37.5887, 44.0352) -> (-37.6208, 44.0352)
  spline S162 degree 2 poles (-37.6208, 44.0352) (-37.6751, 44.0846) (-37.8431, 44.2229) (-37.9641, 44.2896) knots 0 0 0 1 2 2 2
  spline S163 degree 2 poles (-37.9641, 44.2896) (-38.0802, 44.3539) (-38.3544, 44.4354) (-38.5322, 44.4354) knots 0 0 0 1 2 2 2
  spline S164 degree 2 poles (-38.5322, 44.4354) (-38.7273, 44.4354) (-39.0756, 44.2748) (-39.2065, 44.1217) knots 0 0 0 1 2 2 2
  spline S165 degree 2 poles (-39.2065, 44.1217) (-39.335, 43.9661) (-39.4782, 43.4943) (-39.4782, 43.2004) knots 0 0 0 1 2 2 2
  spline S166 degree 2 poles (-39.4782, 43.2004) (-39.4782, 42.8867) (-39.3275, 42.4346) (-39.1966, 42.279) knots 0 0 0 1 2 2 2
  spline S167 degree 2 poles (-39.1966, 42.279) (-39.0682, 42.1284) (-38.7249, 41.9752) (-38.5322, 41.9752) knots 0 0 0 1 2 2 2
  spline S168 degree 2 poles (-38.5322, 41.9752) (-38.3568, 41.9752) (-38.058, 42.0617) (-37.9419, 42.1259) knots 0 0 0 1 2 2 2
  spline S169 degree 2 poles (-37.9419, 42.1259) (-37.8307, 42.1901) (-37.6652, 42.3235) (-37.6183, 42.3704) knots 0 0 0 1 2 2 2
  line L104 (-37.6183, 42.3704) -> (-37.5887, 42.3704)
  line L105 (-37.5887, 42.3704) -> (-37.5887, 41.8863)
  spline S170 degree 2 poles (-37.5887, 41.8863) (-37.6899, 41.8394) (-37.8678, 41.7529) (-37.9937, 41.7134) knots 0 0 0 1 2 2 2
  spline S171 degree 2 poles (-37.9937, 41.7134) (-38.1271, 41.6689) (-38.3544, 41.6245) (-38.5371, 41.6245) knots 0 0 0 1 2 2 2
  line L106 (-37.2107, 41.6788) -> (-37.2107, 44.7268)
  line L107 (-37.2107, 44.7268) -> (-35.3039, 44.7268)
  line L108 (-35.3039, 44.7268) -> (-35.3039, 44.3662)
  line L109 (-35.3039, 44.3662) -> (-36.8057, 44.3662)
  line L110 (-36.8057, 44.3662) -> (-36.8057, 43.5313)
  line L111 (-36.8057, 43.5313) -> (-35.4052, 43.5313)
  line L112 (-35.4052, 43.5313) -> (-35.4052, 43.1707)
  line L113 (-35.4052, 43.1707) -> (-36.8057, 43.1707)
  line L114 (-36.8057, 43.1707) -> (-36.8057, 42.0394)
  line L115 (-36.8057, 42.0394) -> (-35.3039, 42.0394)
  line L116 (-35.3039, 42.0394) -> (-35.3039, 41.6788)
  line L117 (-35.3039, 41.6788) -> (-37.2107, 41.6788)
  line L118 (-32.6783, 41.6788) -> (-33.1327, 41.6788)
  line L119 (-33.1327, 41.6788) -> (-34.4814, 44.3069)
  line L120 (-34.4814, 44.3069) -> (-34.4814, 41.6788)
  line L121 (-34.4814, 41.6788) -> (-34.8593, 41.6788)
  line L122 (-34.8593, 41.6788) -> (-34.8593, 44.7268)
  line L123 (-34.8593, 44.7268) -> (-34.2838, 44.7268)
  line L124 (-34.2838, 44.7268) -> (-33.0562, 42.3136)
  line L125 (-33.0562, 42.3136) -> (-33.0562, 44.7268)
  line L126 (-33.0562, 44.7268) -> (-32.6783, 44.7268)
  line L127 (-32.6783, 44.7268) -> (-32.6783, 41.6788)
  line L128 (-28.8769, 42.7261) -> (-29.24, 42.7261)
  line L129 (-29.24, 42.7261) -> (-29.24, 41.6788)
  line L130 (-29.24, 41.6788) -> (-29.6327, 41.6788)
  line L131 (-29.6327, 41.6788) -> (-29.6327, 42.7261)
  line L132 (-29.6327, 42.7261) -> (-30.9789, 42.7261)
  line L133 (-30.9789, 42.7261) -> (-30.9789, 43.1559)
  line L134 (-30.9789, 43.1559) -> (-29.6154, 44.7268)
  line L135 (-29.6154, 44.7268) -> (-29.24, 44.7268)
  line L136 (-29.24, 44.7268) -> (-29.24, 43.0546)
  line L137 (-29.24, 43.0546) -> (-28.8769, 43.0546)
  line L138 (-28.8769, 43.0546) -> (-28.8769, 42.7261)
  line L139 (-29.6327, 43.0546) -> (-29.6327, 44.2452)
  line L140 (-29.6327, 44.2452) -> (-30.6578, 43.0546)
  line L141 (-30.6578, 43.0546) -> (-29.6327, 43.0546)
  spline S172 degree 2 poles (-26.6539, 43.2028) (-26.6539, 42.3828) (-27.1306, 41.6146) (-27.6271, 41.6146) knots 0 0 0 1 2 2 2
  spline S173 degree 2 poles (-27.6271, 41.6146) (-28.131, 41.6146) (-28.6027, 42.3976) (-28.6027, 43.2004) knots 0 0 0 1 2 2 2
  spline S174 degree 2 poles (-28.6027, 43.2004) (-28.6027, 44.0253) (-28.126, 44.7886) (-27.6271, 44.7886) knots 0 0 0 1 2 2 2
  spline S175 degree 2 poles (-27.6271, 44.7886) (-27.1257, 44.7886) (-26.6539, 43.9982) (-26.6539, 43.2028) knots 0 0 0 1 2 2 2
  spline S176 degree 2 poles (-27.1775, 42.2741) (-27.1183, 42.4248) (-27.0689, 42.8891) (-27.0689, 43.2028) knots 0 0 0 1 2 2 2
  spline S177 degree 2 poles (-27.0689, 43.2028) (-27.0689, 43.5165) (-27.1183, 43.9784) (-27.18, 44.134) knots 0 0 0 1 2 2 2
  spline S178 degree 2 poles (-27.18, 44.134) (-27.2418, 44.2896) (-27.4567, 44.4502) (-27.6271, 44.4502) knots 0 0 0 1 2 2 2
  spline S179 degree 2 poles (-27.6271, 44.4502) (-27.7975, 44.4502) (-28.0173, 44.2896) (-28.0816, 44.1291) knots 0 0 0 1 2 2 2
  spline S180 degree 2 poles (-28.0816, 44.1291) (-28.1433, 43.9735) (-28.1878, 43.4992) (-28.1878, 43.2004) knots 0 0 0 1 2 2 2
  spline S181 degree 2 poles (-28.1878, 43.2004) (-28.1878, 42.8793) (-28.1483, 42.4495) (-28.084, 42.2815) knots 0 0 0 1 2 2 2
  spline S182 degree 2 poles (-28.084, 42.2815) (-28.0248, 42.1234) (-27.8049, 41.953) (-27.6271, 41.953) knots 0 0 0 1 2 2 2
  spline S183 degree 2 poles (-27.6271, 41.953) (-27.4591, 41.953) (-27.2393, 42.1135) (-27.1775, 42.2741) knots 0 0 0 1 2 2 2
  line L142 (-24.3024, 42.7261) -> (-24.6655, 42.7261)
  line L143 (-24.6655, 42.7261) -> (-24.6655, 41.6788)
  line L144 (-24.6655, 41.6788) -> (-25.0583, 41.6788)
  line L145 (-25.0583, 41.6788) -> (-25.0583, 42.7261)
  line L146 (-25.0583, 42.7261) -> (-26.4044, 42.7261)
  line L147 (-26.4044, 42.7261) -> (-26.4044, 43.1559)
  line L148 (-26.4044, 43.1559) -> (-25.041, 44.7268)
  line L149 (-25.041, 44.7268) -> (-24.6655, 44.7268)
  line L150 (-24.6655, 44.7268) -> (-24.6655, 43.0546)
  line L151 (-24.6655, 43.0546) -> (-24.3024, 43.0546)
  line L152 (-24.3024, 43.0546) -> (-24.3024, 42.7261)
  line L153 (-25.0583, 43.0546) -> (-25.0583, 44.2452)
  line L154 (-25.0583, 44.2452) -> (-26.0833, 43.0546)
  line L155 (-26.0833, 43.0546) -> (-25.0583, 43.0546)
  point P0 (1.27, -3.175)
  constraints: 2 other
emboss "Emboss1" sketch "Sketch9" operation cut depth 1.27 direction (-1, 0, 0)
sketch "Sketch10" plane through (-33.9583, 76.2, 1.27) normal (0, 1, 0) x (1, 0, 0)
  arc A0 (17.6871, -21.3512) -> (12.1296, -21.3512) centre (14.9083, -21.3512) ccw projected
  line L0 (12.1296, -26.9088) -> (12.1296, -21.3512) projected
  arc A1 (12.1296, -26.9088) -> (17.6871, -26.9088) centre (14.9083, -26.9088) ccw projected
  line L1 (17.6871, -21.3512) -> (17.6871, -26.9088) projected
  point P0 (33.9583, 1.27)
extrude "Extrusion5" cut sketch "Sketch10" against normal blind 25.4
body "Solid1"
